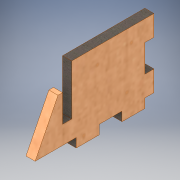
# Autodesk Inventor part: Limiter1
Saved by Autodesk Inventor 2019 (Build 230136000, 136)
## iProperties
Created: 2021-01-03
Part Number: Limiter1
Material: Дерево (вишня)
Document SubType Name: Modeling
Designer: Professional
Density: 0.63 g/cm^3
Appearance: Вишневое дерево — натуральный — со слабым глянцем
Author: Professional
Autodesk Inventor part; units mm, degrees
ref_plane "YZ Plane" through (0, 0, 0) normal (1, 0, 0) x (0, 1, 0)
ref_plane "XZ Plane" through (0, 0, 0) normal (0, 1, 0) x (-1, 0, 0)
ref_plane "XY Plane" through (0, 0, 0) normal (0, 0, 1) x (1, 0, 0)
sketch "Эскиз1" plane through (0, 0, 0) normal (1, 0, 0) x (0, 1, 0)
  line L0 (-4, 15) -> (-4, 5)
  line L1 (-4, 5) -> (0, 5)
  line L2 (0, 5) -> (0, 0)
  line L3 (30, 17) -> (30, 0)
  line L4 (30, 0) -> (0, 0)
  line L5 (-4, -15) -> (-4, -5)
  line L6 (-4, -5) -> (0, -5)
  line L7 (0, -5) -> (0, 0)
  line L8 (30, -17) -> (30, 0)
  line L9 (-4, 15) -> (0, 15)
  line L10 (8, 21) -> (8, 17)
  line L11 (8, 17) -> (30, 17)
  line L12 (-4, -15) -> (0, -15)
  line L13 (0, -15) -> (0, -19)
  line L14 (0, -19) -> (9, -19)
  line L15 (9, -19) -> (9, -15)
  line L16 (9, -15) -> (21, -15)
  line L17 (21, -15) -> (21, -19)
  line L18 (21, -19) -> (30, -19)
  line L19 (30, -19) -> (30, -17)
  line L20 (0, 15) -> (0, 33)
  line L21 (8, 21) -> (20, 21)
  line L22 (20, 21) -> (20, 23)
  line L23 (20, 23) -> (0, 33)
  dimension "d0" = 30
  dimension "d1" = 4
  dimension "d2" = 10
  dimension "d3" = 10
  dimension "d8" = 4
  dimension "d9" = 90
  dimension "d11" = 12
  dimension "d13" = 2
  dimension "d14" = 4
  dimension "d15" = 8
  dimension "d16" = 18
  dimension "d17" = 2
  dimension "d18" = 20
  constraints: 48 end point, 10 perpendicular, 4 point on line, 4 symmetric about line, 3 horizontal, 2 coincident, 2 vertical, 2 vertical alignment, 1 collinear
  measures "d0" distance between parallel lines of L2 L3
  measures "d1" distance of L0.end L1.end
  measures "d2" distance of L0.start L0.end
  measures "d3" diameter of L1 L4
  measures "d8" distance of L12.end L13.end
  measures "d9" angle of L12 L13
  measures "d11" distance between parallel lines of L15 L17
  measures "d13" distance between parallel lines of L9 L11
  measures "d14" distance between parallel lines of L11 L21
  measures "d15" distance between parallel lines of L20 L10
  measures "d16" distance from line of L20.end L9
  measures "d17" distance of L21.end L22.end
  measures "d18" distance between parallel lines of L20 L22
extrude "Выдавливание1" add sketch "Эскиз1" along normal blind 4
